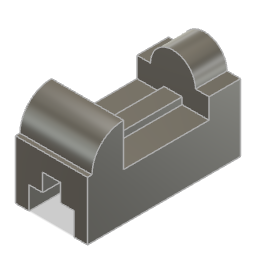
RoboconTask2 v0 (Autodesk Fusion 360 design; units mm, degrees)
Autodesk Fusion 360 part; units mm, degrees
sketch "Sketch1" plane through (0, 0, 0) normal (0, 0, 1) x (1, 0, 0)
  line L0 (-40, -30) -> (-40, 22.5)
  line L1 (-9.9671, 30) -> (10, 30)
  line L2 (40, 22.5) -> (40, -30)
  line L3 (25, -30) -> (25, -4.623)
  line L4 (-25, -4.623) -> (-25, -30)
  line L5 (40, -30) -> (25, -30)
  line L6 (-25, -30) -> (-40, -30)
  line L7 (10, -4.623) -> (10, 15)
  line L8 (10, 15) -> (-9.9671, 15)
  line L9 (-9.9671, 15) -> (-9.9671, -4.623)
  line L10 (10, 22.5) -> (10, 30)
  line L11 (-9.9671, 22.5) -> (-9.9671, 30)
  line L12 (10, 22.5) -> (40, 22.5)
  line L13 (-9.9671, 22.5) -> (-40, 22.5)
  line L14 (25, -4.623) -> (10, -4.623)
  line L15 (-9.9671, -4.623) -> (-25, -4.623)
  constraint horizontal L5
  constraint vertical L0
  constraint horizontal L1
  constraint vertical L2
  constraint vertical L3
  constraint horizontal L14
  constraint vertical L4
  constraint coincident L4.end L5
  constraint collinear L5 L6
  constraint vertical L7
  constraint horizontal L8
  constraint vertical L9
  constraint coincident L9.end L14
  constraint perpendicular L1 L10
  constraint perpendicular L1 L11
  constraint perpendicular L10 L12
  constraint perpendicular L0 L13
  constraint collinear L14 L15
extrude "Extrude1" add sketch "Sketch1" along normal mid plane 170
sketch "Sketch2" plane through (0, 0, 85) normal (0, 0, 1) x (1, 0, 0)
  line L0 (10, 22.5) -> (10, 30)
  line L1 (10, 30) -> (-9.9671, 30)
  line L2 (-9.9671, 30) -> (-9.9671, 22.5)
  line L3 (-9.9671, 22.5) -> (-40, 22.5)
  line L4 (-40, 22.5) -> (-40, -30)
  line L5 (-40, -30) -> (-25, -30)
  line L6 (-25, -30) -> (-25, -4.623)
  line L7 (-25, -4.623) -> (-9.9671, -4.623)
  line L8 (-9.9671, -4.623) -> (-9.9671, 15)
  line L9 (-9.9671, 15) -> (10, 15)
  line L10 (10, 15) -> (10, -4.623)
  line L11 (10, -4.623) -> (25, -4.623)
  line L12 (25, -4.623) -> (25, -30)
  line L13 (25, -30) -> (40, -30)
  line L14 (40, -30) -> (40, 22.5)
  line L15 (40, 22.5) -> (10, 22.5)
  line L16 (-40, 22.5) -> (-40, 35)
  line L17 (-40, 35) -> (40, 35)
  line L18 (40, 35) -> (40, 22.5)
  constraint coincident L3.end L4.start
  constraint perpendicular L3 L16
  constraint perpendicular L16 L17
  constraint coincident L14.end L15.start
  constraint perpendicular L15 L18
extrude "Extrude2" add sketch "Sketch2" against normal blind 40 contours L0 L1 L2 L3 L15 L16 L17 L18
sketch "Sketch3" plane through (40, 0, 0) normal (1, 0, 0) x (0, 0, -1)
  line L0 (85, 22.5) -> (-45, 22.5)
  line L1 (-45, 22.5) -> (-45, 35)
  line L2 (-45, 35) -> (-85, 35)
  line L3 (-85, 35) -> (-85, -30)
  line L4 (-85, -30) -> (85, -30)
  line L5 (85, -30) -> (85, 22.5)
  line L6 (-45, 35) -> (-45, 70)
  arc A0 (-45, 70) -> (-80, 35) centre (-45, 35) ccw
  constraint coincident L1.end L2.start
  constraint perpendicular L2 L6
  constraint coincident L2 A0.end
extrude "Extrude3" add sketch "Sketch3" against normal up to surface (80 mm away) contours L2 L6 A0
sketch "Sketch4" plane through (0, 0, -85) normal (0, 0, -1) x (-1, 0, 0)
  line L0 (-10, 30) -> (-10, 22.5)
  line L1 (-10, 22.5) -> (-40, 22.5)
  line L2 (-40, 22.5) -> (-40, -30)
  line L3 (-40, -30) -> (-25, -30)
  line L4 (-25, -30) -> (-25, -4.623)
  line L5 (-25, -4.623) -> (-10, -4.623)
  line L6 (-10, -4.623) -> (-10, 15)
  line L7 (-10, 15) -> (9.9671, 15)
  line L8 (9.9671, 15) -> (9.9671, -4.623)
  line L9 (9.9671, -4.623) -> (25, -4.623)
  line L10 (25, -4.623) -> (25, -30)
  line L11 (25, -30) -> (40, -30)
  line L12 (40, -30) -> (40, 22.5)
  line L13 (40, 22.5) -> (9.9671, 22.5)
  line L14 (9.9671, 22.5) -> (9.9671, 30)
  line L15 (9.9671, 30) -> (-10, 30)
  line L16 (-40, 22.5) -> (-40, 45)
  line L17 (40, 45) -> (40, 22.5)
  arc A0 (25, 45) -> (-25, 45) centre (0, 45) ccw
  line L18 (-40, 45) -> (-25, 45)
  line L19 (25, 45) -> (40, 45)
  constraint coincident L1.end L2.start
  constraint perpendicular L1 L16
  constraint perpendicular L16 L18
  constraint coincident L12.end L13.start
  constraint coincident A0.start L18
  constraint collinear L18 L19
  constraint coincident A0.centre L18
extrude "Extrude4" add sketch "Sketch4" against normal blind 35 contours L0 L1 L13 L14 L15 L16 L17 A0 L18 L19
